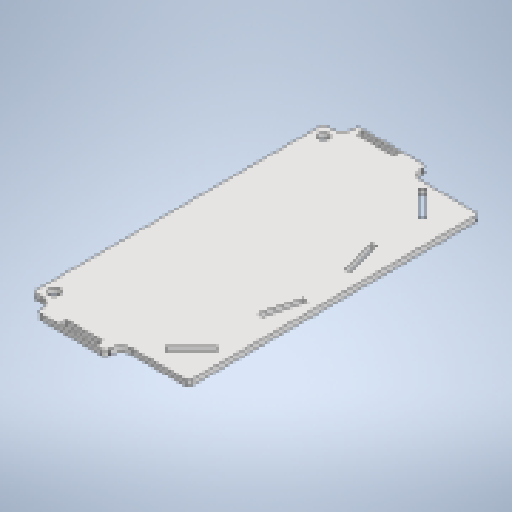
# Autodesk Inventor part: pcb_pre
Saved by Autodesk Inventor 2023 (Build 270158000, 158)
## iProperties
Created: 2025-01-11
Part Number: pcb_pre
Material: Ogólny
Document SubType Name: Modeling
Designer: kamil
Density: 1 g/cm^3
Appearance: Domyślna
Author: kamil
Autodesk Inventor part; units mm, degrees
ref_plane "YZ Plane" through (0, 0, 0) normal (1, 0, 0) x (0, 1, 0)
ref_plane "XZ Plane" through (0, 0, 0) normal (0, 1, 0) x (-1, 0, 0)
ref_plane "XY Plane" through (0, 0, 0) normal (0, 0, 1) x (1, 0, 0)
sketch "Szkic1" plane through (0, 0, 0) normal (0, 1, 0) x (-1, 0, 0)
  line L0 (0, 0) -> (-45, 0)
  line L1 (-45, 0) -> (-45, -84)
  line L2 (-45, -84) -> (0, -84)
  line L3 (0, -84) -> (0, 0)
  dimension "d0" = 45
  dimension "d1" = 84
  constraints: 8 end point, 2 parallel, 1 horizontal, 1 perpendicular
  measures "d0" distance of L2.end L1.end
  measures "d1" distance of L1.end L0.end
extrude "Wyciągnięcie proste1" add sketch "Szkic1" along normal blind 1.6
sketch "Szkic2" plane through (0, 0, 0) normal (0, -1, 0) x (1, 0, 0)
  line L0 (5, 5) -> (5, 4.5) projected
  line L1 (25.8844, 4.5) -> (25.8844, 5) projected
  line L2 (25.8844, -88.5) -> (25.8844, -89) projected
  line L3 (5, -89) -> (5, -88.5) projected
  line L4 (45, 0) -> (45, -84) projected
  line L5 (0, 0) -> (45, 0) projected
  line L6 (0, -84) -> (0, 0) projected
  line L7 (45, -84) -> (0, -84) projected
  line L8 (25.8844, 5) -> (5, 5)
  line L9 (5, 5) -> (5, -3.0099)
  line L10 (5, -3.0099) -> (25.8844, -3.0099)
  line L11 (25.8844, -3.0099) -> (25.8844, 5)
  line L12 (25.8844, -89) -> (5, -89)
  line L13 (5, -89) -> (5, -80.3715)
  line L14 (5, -80.3715) -> (25.8844, -80.3715)
  line L15 (25.8844, -80.3715) -> (25.8844, -89)
  line L16 (25.3844, -88.5) -> (5.5, -88.5)
  line L17 (5.5, -88.5) -> (5.5, -80.8715)
  line L18 (5.5, -80.8715) -> (25.3844, -80.8715)
  line L19 (25.3844, -80.8715) -> (25.3844, -88.5)
  line L20 (25.3844, 4.5) -> (5.5, 4.5)
  line L21 (5.5, 4.5) -> (5.5, -2.5099)
  line L22 (5.5, -2.5099) -> (25.3844, -2.5099)
  line L23 (25.3844, -2.5099) -> (25.3844, 4.5)
  point P0 (25.3844, -84)
  point P1 (5.5, -84)
  point P2 (5.5, 0)
  point P3 (25.3844, 0)
  dimension "d4" = 0.5
  dimension "d5" = 0.5
  constraints: 32 end point, 8 parallel, 4 perpendicular, 2 horizontal, 1 point on line, 6 other
  measures "d4" distance between parallel lines of L15 L19
  measures "d5" distance between parallel lines of L11 L23
extrude "Wyciągnięcie proste2" add sketch "Szkic2" against normal up to surface (1.6 mm away) contours L21 L20 L23 L5 | L7 L19 L16 L17
fillet "Zaokrąglenie1" radius 3 4 edges at (5.5, 0.8, -84) (25.3844, 0.8, -84) (5.5, 0.8, 0) (25.3844, 0.8, 0)
fillet "Zaokrąglenie2" radius 1 8 edges at (25.3844, 0.8, -88.5) (5.5, 0.8, -88.5) (5.5, 0.8, 4.5) (25.3844, 0.8, 4.5) (45, 0.8, 0) (45, 0.8, -84) (0, 0.8, -84) (0, 0.8, 0)
sketch "Szkic3" plane through (0, 0, 0) normal (0, -1, 0) x (1, 0, 0)
  line L0 (18.2, -87.9) -> (18.2, -86.3) projected
  line L1 (7.5, -87.9) -> (7.5, -86.3) projected
  line L2 (18.2, -87.9) -> (7.5, -87.9) projected
  line L3 (7.5, -86.3) -> (18.2, -86.3) projected
  line L4 (22.5, 2.3) -> (11.8, 2.3) projected
  line L5 (11.8, 3.9) -> (11.8, 2.3) projected
  line L6 (11.8, 3.9) -> (22.5, 3.9) projected
  line L7 (22.5, 3.9) -> (22.5, 2.3) projected
  line L8 (34.0305, -4.1816) -> (32.8991, -5.313) projected
  line L9 (40.4652, -12.879) -> (32.8991, -5.313) projected
  line L10 (34.0305, -4.1816) -> (41.5966, -11.7477) projected
  line L11 (41.5966, -11.7477) -> (40.4652, -12.879) projected
  line L12 (42.2206, -37.1194) -> (40.6751, -37.5335) projected
  line L13 (40.6751, -37.5335) -> (37.9058, -27.1981) projected
  line L14 (39.4513, -26.784) -> (42.2206, -37.1194) projected
  line L15 (39.4513, -26.784) -> (37.9058, -27.1981) projected
  line L16 (38.3383, -61.3695) -> (36.7929, -60.9554) projected
  line L17 (36.7929, -60.9554) -> (39.5622, -50.62) projected
  line L18 (41.1077, -51.0341) -> (38.3383, -61.3695) projected
  line L19 (41.1077, -51.0341) -> (39.5622, -50.62) projected
  line L20 (30.99, -82.8589) -> (29.8586, -81.7276) projected
  line L21 (29.8586, -81.7276) -> (37.4246, -74.1615) projected
  line L22 (38.556, -75.2929) -> (30.99, -82.8589) projected
  line L23 (38.556, -75.2929) -> (37.4246, -74.1615) projected
  circle A0 centre (3, -81) radius 1.55
  circle A1 centre (3, -3) radius 1.55
  arc A2 (1, 0) -> (0, -1) centre (1, -1) ccw projected
  line L24 (0, -83) -> (0, -1) projected
  arc A3 (0, -83) -> (1, -84) centre (1, -83) ccw projected
  line L25 (2.5, -84) -> (1, -84) projected
  arc A4 (5.5, -87) -> (2.5, -84) centre (2.5, -87) ccw projected
  line L26 (5.5, -87) -> (5.5, -87.5) projected
  arc A5 (5.5, -87.5) -> (6.5, -88.5) centre (6.5, -87.5) ccw projected
  line L27 (6.5, -88.5) -> (24.3844, -88.5) projected
  arc A6 (24.3844, -88.5) -> (25.3844, -87.5) centre (24.3844, -87.5) ccw projected
  line L28 (25.3844, -87.5) -> (25.3844, -87) projected
  arc A7 (28.3844, -84) -> (25.3844, -87) centre (28.3844, -87) ccw projected
  line L29 (44, -84) -> (28.3844, -84) projected
  arc A8 (44, -84) -> (45, -83) centre (44, -83) ccw projected
  line L30 (45, -1) -> (45, -83) projected
  arc A9 (45, -1) -> (44, 0) centre (44, -1) ccw projected
  line L31 (28.3844, 0) -> (44, 0) projected
  arc A10 (25.3844, 3) -> (28.3844, 0) centre (28.3844, 3) ccw projected
  line L32 (25.3844, 3) -> (25.3844, 3.5) projected
  arc A11 (25.3844, 3.5) -> (24.3844, 4.5) centre (24.3844, 3.5) ccw projected
  line L33 (24.3844, 4.5) -> (6.5, 4.5) projected
  arc A12 (6.5, 4.5) -> (5.5, 3.5) centre (6.5, 3.5) ccw projected
  line L34 (5.5, 3.5) -> (5.5, 3) projected
  arc A13 (2.5, 0) -> (5.5, 3) centre (2.5, 3) ccw projected
  line L35 (1, 0) -> (2.5, 0) projected
  point P0 (0, 0)
  point P1 (1.75, -84)
  dimension "d10" = 3.1
  dimension "d11" = 3.1
  dimension "d12" = 3
  dimension "d13" = 3
  dimension "d14" = 3
  dimension "d15" = 3
  constraints: 2 centre point, 1 midpoint
  measures "d10" diameter of A0
  measures "d11" diameter of A1
  measures "d12" distance from line of L24 A1.centre
  measures "d13" distance from line of A1.centre L35
  measures "d14" distance from line of A0.centre L24
  measures "d15" vertical distance of point (1.75, -84) A0.centre
extrude "Wyciągnięcie proste3" cut sketch "Szkic3" against normal through all contours L2 L1 L3 L0 | L4 L5 L6 L7 | L10 L11 L9 L8 | L12 L13 L15 L14 | L16 L17 L19 L18 | L20 L21 L23 L22 | A0 | A1
